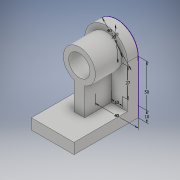
# Autodesk Inventor part: A
Saved by Autodesk Inventor 2018 (Build 220112000, 112)
## iProperties
Created: 2017-09-30
Part Number: A
Material: Generic
Document SubType Name: Modeling
Designer: Soichi
Density: 1 g/cm^3
Appearance: Default
Author: Soichi
Autodesk Inventor part; units mm, degrees
ref_plane "YZ Plane" through (0, 0, 0) normal (1, 0, 0) x (0, 1, 0)
ref_plane "XZ Plane" through (0, 0, 0) normal (0, 1, 0) x (-1, 0, 0)
ref_plane "XY Plane" through (0, 0, 0) normal (0, 0, 1) x (1, 0, 0)
sketch "Sketch1" plane through (0, 0, 0) normal (0, 0, 1) x (1, 0, 0)
  circle A0 centre (0, 0) radius 10
  circle A1 centre (0, 0) radius 15
  circle A2 centre (0, 0) radius 20
  line L0 (-20, 0) -> (20, 0)
  line L1 (20, 0) -> (20, -50)
  line L2 (20, -50) -> (-20, -50)
  line L3 (-20, -50) -> (-20, 0)
  line L4 (-20, -40) -> (20, -40)
  line L5 (20, -40) -> (20, -50)
  line L6 (20, -50) -> (-20, -50)
  line L7 (-20, -50) -> (-20, -40)
  line L8 (-5, -13) -> (5, -13)
  line L9 (5, -13) -> (5, -40)
  line L10 (5, -40) -> (-5, -40)
  line L11 (-5, -40) -> (-5, -13)
  point P0 (0, -50)
  point P1 (0, -40)
  dimension "d0" = 20
  dimension "d1" = 30
  dimension "d2" = 40
  dimension "d3" = 40
  dimension "d4" = 50
  dimension "d5" = 40
  dimension "d6" = 10
  dimension "d7" = 10
  dimension "d8" = 27
  constraints: 24 end point, 6 parallel, 5 midpoint, 4 coincident, 3 centre point, 3 horizontal, 3 perpendicular
  measures "d0" diameter of A0
  measures "d1" diameter of A1
  measures "d2" diameter of A2
  measures "d3" distance of L1.end L2.end
  measures "d4" distance of L0.end L1.end
  measures "d5" distance of L5.end L6.end
  measures "d6" distance of L4.end L5.end
  measures "d7" distance of L9.end L10.end
  measures "d8" distance of L8.end L9.end
extrude "Extrusion1" add sketch "Sketch1" along normal blind 35 contours L0 A1 L9 L8 L11 A0 | A0 L0 A1 | L9 A2 L11 A1 | A1 L11 L8 L9 | L9 L4 L11 A2
extrude "Extrusion2" add sketch "Sketch1" along normal blind 10 contours L0 A0 | A0 L0 | L0 A2 L9 A1 | A1 L0 A2 | A1 L11 A2 L0 | L1 L4 L9 A2 | A2 L11 L4 L3
extrude "Extrusion3" add sketch "Sketch1" along normal blind 60 contours L1 L2 L3 L4
body "Solid1"
